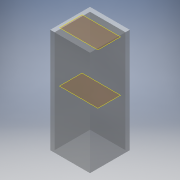
# Autodesk Inventor part: Cuvette
Saved by Autodesk Inventor 2019 (Build 230136000, 136)
## iProperties
Created: 2019-09-25
Part Number: Cuvette
Material: Generic
Document SubType Name: Modeling
Designer: voigt
Density: 1 g/cm^3
Appearance: Clear
Author: voigt
Autodesk Inventor part; units mm, degrees
ref_plane "YZ Plane" through (0, 0, 0) normal (1, 0, 0) x (0, 1, 0)
ref_plane "XZ Plane" through (0, 0, 0) normal (0, 1, 0) x (-1, 0, 0)
ref_plane "XY Plane" through (0, 0, 0) normal (0, 0, 1) x (1, 0, 0)
ref_plane "Work Plane1" through (37.4102, 3.6005, -54.5986) normal (0, 1, 0) x (-1, 0, 0)
ref_plane "Work Plane2" through (37.4102, 122.9805, -54.5986) normal (0, 1, 0) x (-1, 0, 0)
sketch "Sketch2" plane through (37.4102, 122.9805, -54.5986) normal (0, 1, 0) x (-1, 0, 0)
  line L0 (1.8502, -16.6863) -> (-81.9698, -16.6863)
  line L1 (-81.9698, -16.6863) -> (-81.9698, 67.1337)
  line L2 (-81.9698, 67.1337) -> (1.8502, 67.1337)
  line L3 (1.8502, 67.1337) -> (1.8502, -16.6863)
  line L4 (37.4102, -40.5623) -> (37.4102, 91.0097) construction
  line L5 (-111.9418, 54.5986) -> (62.3022, 54.5986) construction
  line L6 (6.9302, -21.7663) -> (-87.0498, -21.7663)
  line L7 (-87.0498, -21.7663) -> (-87.0498, 72.2137)
  line L8 (-87.0498, 72.2137) -> (6.9302, 72.2137)
  line L9 (6.9302, 72.2137) -> (6.9302, -21.7663)
  point P0 (37.4102, 54.5986)
  dimension "d1" = 83.82
  dimension "d2" = 83.82
  dimension "d3" = 35.56
  dimension "d4" = 12.5351
  dimension "d5" = 5.08
  dimension "d6" = 5.08
  dimension "d7" = 5.08
  dimension "d8" = 5.08
  constraints: 16 end point, 4 parallel, 2 horizontal, 2 perpendicular
  measures "d1" distance of L1.end L2.end
  measures "d2" distance of L0.end L1.end
  measures "d3" distance between parallel lines of L4 L3
  measures "d4" distance between parallel lines of L5 L2
  measures "d5" distance between parallel lines of L6 L0
  measures "d6" distance between parallel lines of L3 L9
  measures "d7" distance between parallel lines of L2 L8
  measures "d8" distance between parallel lines of L1 L7
extrude "Extrusion1" add sketch "Sketch2" against normal blind 254
sketch "Sketch3" plane through (37.4102, 122.9805, -54.5986) normal (0, 1, 0) x (1, 0, 0)
  line L0 (-6.9302, 21.7663) -> (87.0498, 21.7663) projected
  line L1 (-6.9302, -72.2137) -> (-6.9302, 21.7663) projected
  line L2 (87.0498, 21.7663) -> (87.0498, -72.2137) projected
  line L3 (87.0498, -72.2137) -> (-6.9302, -72.2137) projected
  point P0 (-37.4102, -54.5986)
extrude "Extrusion2" add sketch "Sketch3" along normal blind 5.08
body "Solid1"
